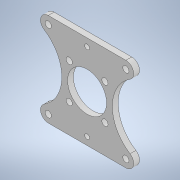
# Autodesk Inventor part: 関節3_555側_モータマウント
Saved by Autodesk Inventor 2021 (Build 250183000, 183)
## iProperties
Created: 2022-01-31
Part Number: 関節3_555側_モータマウント
Material: 一般
Document SubType Name: Modeling
Designer: hirohumi
Density: 1 g/cm^3
Appearance: 既定
Author: hirohumi
Autodesk Inventor part; units mm, degrees
ref_plane "YZ Plane" through (0, 0, 0) normal (1, 0, 0) x (0, 1, 0)
ref_plane "XZ Plane" through (0, 0, 0) normal (0, 1, 0) x (-1, 0, 0)
ref_plane "XY Plane" through (0, 0, 0) normal (0, 0, 1) x (1, 0, 0)
sketch "スケッチ1" plane through (0, 0, 0) normal (0, 0, 1) x (1, 0, 0)
  circle A0 centre (0, 0) radius 10.05
  line L0 (20, 20) -> (-20, 20) construction
  line L1 (-20, 20) -> (-20, -20) construction
  line L2 (-20, -20) -> (20, -20) construction
  line L3 (20, -20) -> (20, 20) construction
  line L4 (20, 20) -> (-20, -20) construction
  line L5 (-20, 20) -> (20, -20) construction
  circle A1 centre (-20, 20) radius 1.6
  circle A2 centre (20, 20) radius 1.6
  circle A3 centre (20, -20) radius 1.6
  circle A4 centre (-20, -20) radius 1.6
  circle A5 centre (0, 0) radius 13 construction
  circle A6 centre (9.1924, 9.1924) radius 1.6
  circle A7 centre (-9.1924, 9.1924) radius 1.6
  circle A8 centre (-9.1924, -9.1924) radius 1.6
  circle A9 centre (9.1924, -9.1924) radius 1.6
  arc A10 (-20, 24) -> (-22.142, 16.6219) centre (-20, 20) ccw
  arc A11 (-22.142, -16.6219) -> (-20, -24) centre (-20, -20) ccw
  arc A12 (20, -24) -> (22.142, -16.6219) centre (20, -20) ccw
  arc A13 (22.142, 16.6219) -> (20, 24) centre (20, 20) ccw
  arc A14 (22.142, 16.6219) -> (22.142, -16.6219) centre (32.6818, 0) ccw
  arc A15 (-22.142, -16.6219) -> (-22.142, 16.6219) centre (-32.6818, 0) ccw
  circle A16 centre (0, 20) radius 1.25
  circle A17 centre (0, -20) radius 1.25
  line L6 (-20, 24) -> (20, 24)
  line L7 (-20, -24) -> (20, -24)
  dimension "d0" = 20.1
  dimension "d1" = 40
  dimension "d2" = 40
  dimension "d3" = 3.2
  dimension "d4" = 3.2
  dimension "d5" = 3.2
  dimension "d6" = 3.2
  dimension "d7" = 26
  dimension "d8" = 3.2
  dimension "d9" = 3.2
  dimension "d10" = 3.2
  dimension "d11" = 3.2
  dimension "d12" = 4
  dimension "d13" = 4
  dimension "d14" = 4
  dimension "d15" = 4
  dimension "d18" = 2.5
  dimension "d19" = 2.5
  constraints: 18 centre point, 16 end point, 16 point on circle, 10 coincident, 8 tangent, 4 midpoint, 4 point on line, 3 parallel, 2 horizontal, 1 perpendicular
  measures "d0" diameter of A0
  measures "d1" distance of L2.end L1.end
  measures "d2" distance of L1.end L0.end
  measures "d3" diameter of A1
  measures "d4" diameter of A2
  measures "d5" diameter of A3
  measures "d6" diameter of A4
  measures "d7" diameter of A5
  measures "d8" diameter of A6
  measures "d9" diameter of A7
  measures "d10" diameter of A8
  measures "d11" diameter of A9
  measures "d12" radius of A10
  measures "d13" radius of A11
  measures "d14" radius of A12
  measures "d15" radius of A13
  measures "d18" diameter of A16
  measures "d19" diameter of A17
extrude "押し出し1" add sketch "スケッチ1" along normal blind 3
